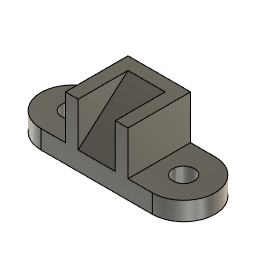
Lab 3 A2 (Autodesk Fusion 360 design; units mm, degrees)
Autodesk Fusion 360 part; units mm, degrees
sketch "Sketch1" plane through (0, 0, 0) normal (0, 0, 1) x (1, 0, 0)
  line L0 (57, -32) -> (-57, -32)
  line L1 (-57, 32) -> (57, 32)
  circle A0 centre (-57, 0) radius 11
  circle A1 centre (57, 0) radius 11
  line L2 (-32, -32) -> (-32, 32)
  line L3 (32, 32) -> (32, -32)
  line L4 (-19, -32) -> (-19, 19)
  line L5 (19, -32) -> (19, 19)
  line L6 (-19, 19) -> (19, 19)
  arc A2 (-29.6806, 16.6628) -> (-32, 19.975) centre (-57, 0) ccw
  line L7 (32, -17.9649) -> (29.6806, -16.6628) construction
  line L8 (-29.6806, 16.6628) -> (-32, 17.9649) construction
  line L9 (-32, -17.9649) -> (-29.6806, -16.6628) construction
  line L10 (29.6806, 16.6628) -> (32, 17.9649) construction
  arc A3 (-57, 32) -> (-57, -32) centre (-57, 0) ccw
  arc A4 (-32, -19.975) -> (-29.6806, -16.6628) centre (-57, 0) ccw
  arc A5 (57, -32) -> (57, 32) centre (57, 0) ccw
  arc A6 (32, 19.975) -> (29.6806, 16.6628) centre (57, 0) ccw
  arc A7 (29.6806, -16.6628) -> (32, -19.975) centre (57, 0) ccw
  dimension "d1" = 114
  dimension "d2" = 64
  dimension "d3" = 64
  dimension "d4" = 22
  dimension "d5" = 64
  dimension "d6" = 22
  dimension "d7" = 64
  dimension "d9" = 13
  dimension "d10" = 13
  dimension "d11" = 13
  constraint parallel L0 L1
  constraint horizontal L0
  constraint coincident origin L7
  constraint coincident origin L9
  constraint concentric A0 A2
  constraint concentric A1 A6
  constraint coincident L0 L2.start
  constraint coincident L1 L2.end
  constraint perpendicular L1 L2
  constraint coincident L1 L3.start
  constraint coincident L0 L3.end
  constraint perpendicular L0 L3
  constraint coincident L0 L4.start
  constraint perpendicular L0 L4
  constraint coincident L0 L5.start
  constraint perpendicular L0 L5
  constraint perpendicular L5 L6
  constraint coincident A2.start L7
  constraint coincident L2 A2.end
  constraint concentric A2 A3
  constraint coincident L2 L8.end
  constraint collinear L7 L8
  constraint coincident L3 A6.start
  constraint coincident L3 L10.end
  constraint collinear L9 L10
  constraint coincident L7.end A6
  constraint coincident L3 L7.start
  constraint coincident L2 L9.start
  constraint coincident L2 A4.start
  constraint concentric A3 A4
  constraint coincident L3 A7.end
  constraint concentric A5 A6
  constraint concentric A6 A7
  measures "d1" distance of L1.start L1.end
  measures "d2" distance of L0.end L1.start
  measures "d3" diameter of A2
  measures "d4" diameter of A0
  measures "d5" diameter of A6
  measures "d6" diameter of A1
  measures "d7" distance of L2 L3
  measures "d9" distance of L2 L4
  measures "d10" distance of L3 L5
  measures "d11" distance of L1 L6
sketch "Sketch2" plane through (0, 0, 0) normal (1, 0, 0) x (0, 1, 0)
  line L0 (-32, 0) -> (32, 0)
  line L1 (32, 0) -> (32, 64)
  line L2 (32, 64) -> (-32, 64)
  line L3 (-32, 64) -> (-32, 0)
  line L4 (32, 64) -> (19, 64)
  line L5 (-32, 0) -> (-32, 19)
  line L6 (-32, 19) -> (19, 64)
  line L7 (19, 64) -> (19, 19)
  line L8 (19, 19) -> (-32, 19)
  dimension "d12" = 64
  dimension "d13" = 64
  dimension "d14" = 13
  dimension "d15" = 19
  constraint horizontal L0
  constraint vertical L1
  constraint horizontal L2
  constraint vertical L3
  constraint perpendicular L1 L4
  constraint perpendicular L0 L5
  constraint perpendicular L2 L7
  constraint perpendicular L3 L8
  measures "d12" distance of L0.start L0.end
  measures "d13" distance of L0.start L2.end
  measures "d14" distance of L1.end L4.end
  measures "d15" distance of L0.start L5.end
extrude "Extrude1" add sketch "Sketch2" along normal mid plane 38 contours L6 L7 L8 makes body 1
extrude "Extrude2" add sketch "Sketch1" along normal blind 19 contours L0 L1 L3 A5 | L0 L4 L5 L6 | L0 L1 L2 A3 bodies 1 makes body 2 at (-46.8333, 24.5088, 0) makes body 3 at (46.8333, 24.5088, 0)
extrude "Extrude3" add sketch "Sketch1" along normal blind 64 contours L0 L1 L2 L3 L4 L5 L6 bodies 1 2 3
